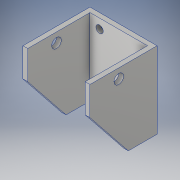
# Autodesk Inventor part: CAR_016_TensionerMount
Saved by Autodesk Inventor 2018 (Build 220112000, 112)
## iProperties
Created: 2020-02-01
Part Number: CAR_016_TensionerMount
Material: Aluminum 6061
Document SubType Name: Modeling
Designer: user
Mass: 47.3797 g
Surface Area: 123.493 cm^2
Volume: 17.548 cm^3
Density: 2.7 g/cm^3
Appearance: Aluminum - Flat
Author: user
Autodesk Inventor part; units mm, degrees
ref_plane "YZ Plane" through (0, 0, 0) normal (1, 0, 0) x (0, 1, 0)
ref_plane "XZ Plane" through (0, 0, 0) normal (0, 1, 0) x (-1, 0, 0)
ref_plane "XY Plane" through (0, 0, 0) normal (0, 0, 1) x (1, 0, 0)
sketch "Sketch1" plane through (0, 0, 0) normal (0, 1, 0) x (-1, 0, 0)
  line L0 (0, 0) -> (44.45, 0)
  line L1 (44.45, 0) -> (44.45, -44.45)
  line L2 (44.45, -44.45) -> (0, -44.45)
  line L3 (0, -44.45) -> (0, 0)
  line L4 (41.275, -41.275) -> (41.275, -3.175)
  line L5 (41.275, -3.175) -> (3.175, -3.175)
  line L6 (3.175, -3.175) -> (3.175, -41.275)
  line L7 (3.175, -41.275) -> (41.275, -41.275)
  line L8 (41.275, -3.175) -> (41.275, 0)
  line L9 (3.175, -3.175) -> (3.175, 0)
  dimension "d0" = 3.175
  dimension "d1" = 44.45
  constraints: 20 end point, 4 parallel, 4 perpendicular, 2 point on line, 1 horizontal, 1 vertical, 3 other
  measures "d0" distance between parallel lines of L1 L4
  measures "d1" distance of L1.end L2.end
extrude "Extrusion1" add sketch "Sketch1" along normal blind 50.8 contours L0 L9 L6 L7 L4 L8 L1 L2 L3
sketch "Sketch2" plane through (0, 0, 0) normal (1, 0, 0) x (0, 0, -1)
  line L0 (0, 50.8) -> (44.45, 50.8) projected
  line L1 (0, 0) -> (0, 50.8) projected
  line L2 (44.45, 0) -> (44.45, 50.8) projected
  point P0 (19.05, 44.45)
  dimension "d11" = 6.35
  dimension "d13" = 25.4
  measures "d11" distance from line of L0 point (19.05, 44.45)
  measures "d13" distance from line of L2 point (19.05, 44.45)
hole "Hole1" at (0, 44.45, -19.05) direction (-1, 0, 0) diameter 6.35 end through all
sketch "Sketch3" plane through (0, 0, -44.45) normal (0, 0, -1) x (-1, 0, 0)
  line L0 (16.2052, 86.1658) -> (16.2052, -32.4239) construction
  line L1 (0, 0) -> (0, 50.8) construction
  line L2 (44.45, 0) -> (44.45, 50.8) construction
  line L3 (0, 50.8) -> (44.45, 50.8) construction
  line L4 (0, 0) -> (44.45, 0) projected
  point P0 (34.925, 44.45)
  point P1 (34.925, 6.35)
  point P2 (22.5552, 6.35)
  point P3 (22.5552, 44.45)
  dimension "d14" = 16.2052
  dimension "d17" = 6.35
  dimension "d18" = 6.35
  dimension "d19" = 6.35
  dimension "d30" = 6.35
  dimension "d31" = 9.525
  dimension "d32" = 9.525
  dimension "d33" = 6.35
  dimension "d34" = 6.35
  constraints: 2 end point, 1 vertical
  measures "d14" distance between parallel lines of L0 L1
  measures "d17" distance from line of L3 point (34.925, 44.45)
  measures "d18" distance from line of L3 point (22.555, 44.45)
  measures "d19" distance from line of L4 point (22.555, 6.35)
  measures "d30" distance from line of L4 point (34.925, 6.35)
  measures "d31" distance from line of L2 point (34.925, 6.35)
  measures "d32" distance from line of L2 point (34.925, 44.45)
  measures "d33" distance from line of L0 point (22.555, 44.45)
  measures "d34" distance from line of L0 point (22.555, 6.35)
hole "Hole2" at (-34.925, 44.45, -44.45) at (-34.925, 6.35, -44.45) at (-22.5552, 6.35, -44.45) direction (0, 0, 1) diameter 4.826 end through all
sketch "Sketch4" plane through (-44.45, 0, -44.45) normal (-1, 0, 0) x (0, 0, 1)
  line L0 (19.05, 0) -> (44.45, 31.75)
  circle A0 centre (25.4, 44.45) radius 3.175 projected
  line L1 (0, 0) -> (44.45, 0) projected
  line L2 (44.45, 0) -> (44.45, 50.8) projected
  line L3 (0, 50.8) -> (44.45, 50.8) projected
  line L4 (0, 0) -> (0, 50.8) projected
  point P0 (44.45, 0)
  dimension "d35" = 19.05
  dimension "d36" = 25.4
  constraints: 2 end point, 2 point on line
  measures "d35" distance from line of L3 L0.end
  measures "d36" distance from line of L2 L0.start
extrude "Extrusion2" cut sketch "Sketch4" against normal blind 152.4 contours L0 L2 L1
equation "\"d18\" = d17"
equation "\"d19\" = d18"
equation "\"d30\" = d17"
equation "\"d32\" = d31"
equation "\"d34\" = d33"
body "Solid1"
